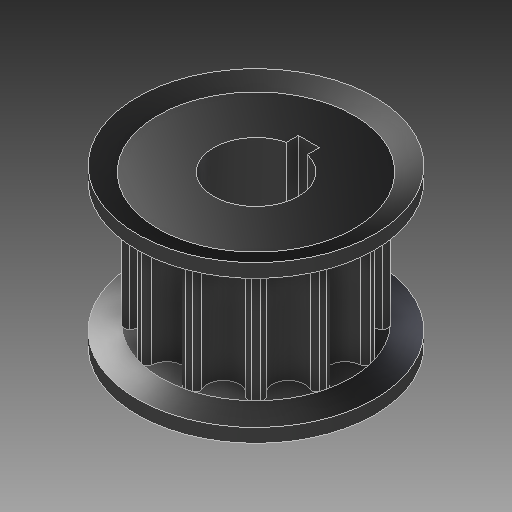
# Autodesk Inventor part: Timing Pulleys
Saved by Autodesk Inventor 2023 (Build 270158000, 158)
## iProperties
Created: 2020-11-14
Material: Nylon 6/6
Document SubType Name: Modeling
Density: 1.13 g/cm^3
Appearance: Glossy - Black
Mass: 24.0165 g
Surface Area: 135.444 cm^2
Volume: 21.2535 cm^3
Revision Number: 0
Autodesk Inventor part; units mm, degrees
ref_plane "YZ Plane" through (0, 0, 0) normal (1, 0, 0) x (0, 1, 0)
ref_plane "XZ Plane" through (0, 0, 0) normal (0, 1, 0) x (-1, 0, 0)
ref_plane "XY Plane" through (0, 0, 0) normal (0, 0, 1) x (1, 0, 0)
sketch "Sketch1" plane through (0, 0, 0) normal (0, 1, 0) x (-1, 0, 0)
  circle A0 centre (0, 0) radius 8.9778
  dimension "d0" = 17.9556
  constraints: 1 centre point, 1 coincident
  measures "d0" diameter of A0
extrude "Extrusion1" add sketch "Sketch1" along normal mid plane 11
sketch "Sketch10" plane through (0, -5.5, 0) normal (0, -1, 0) x (1, 0, 0)
  circle A0 centre (0, 0) radius 8.9778 projected
  circle A1 centre (0, 0) radius 6.9178 construction
  arc A2 (1.5221, -8.3486) -> (-1.5221, -8.3486) centre (0, -8.4428) ccw
  arc A3 (-2.0494, -8.7407) -> (-1.5221, -8.3486) centre (-1.9513, -8.3221) ccw
  line L0 (0, 0) -> (0, -17.4745) construction
  line L1 (0, 0) -> (-8.9342, -15.4745) construction
  circle A4 centre (0, 0) radius 8.9778 projected
  arc A5 (1.5221, -8.3486) -> (2.0494, -8.7407) centre (1.9513, -8.3221) ccw
  point P0 (-2.0494, -8.7407)
  dimension "d62" = 2.06
  dimension "d63" = 3.05
  dimension "d64" = 0.86
  dimension "d65" = 30
  constraints: 8 point on circle, 4 centre point, 4 end point, 3 tangent, 1 symmetric about line, 1 vertical, 1 vertical alignment, 1 other
  measures "d62" radial gap between concentric circles of A0 A1
  measures "d63" diameter of A2
  measures "d64" diameter of A3
  measures "d65" angle of L0 L1
extrude "HTD 5mm Profile" cut sketch "Sketch10" against normal blind 25.4 contours A3 A2 A5 A0 picked at (0.0589, -8.2769)
sketch "Sketch2" plane through (0, 5.5, 0) normal (0, 1, 0) x (1, 0, 0)
  arc A0 (-2.0494, 8.7407) -> (2.0494, 8.7407) centre (0, 0) ccw projected
  arc A1 (-8.8102, -1.0082) -> (-8.9151, -1.0594) centre (-8.7336, -1.298) ccw
  arc A2 (-8.5536, -0.9436) -> (-8.5536, 0.9436) centre (-8.7797, 0) ccw
  arc A3 (-8.9151, 1.0594) -> (-8.8102, 1.0082) centre (-8.7336, 1.298) ccw
  line L0 (0, 0) -> (-21.2101, 0) construction
  arc A4 (-8.5536, -0.9436) -> (-8.8102, -1.0082) centre (-5.8906, -12.059) ccw
  arc A5 (-8.8102, 1.0082) -> (-8.5536, 0.9436) centre (-5.8906, 12.059) ccw
  line L1 (0, 0) -> (0, 6.3397) construction
  line L2 (-8.9778, 0) -> (-8.9778, -190.5824) construction
  arc A6 (-8.9151, 1.0594) -> (-8.9151, -1.0594) centre (0, 0) ccw
  dimension "d3" = 0.9703
  dimension "d5" = 0.2997
  dimension "d7" = 11.43
  dimension "d9" = 7.8094
  dimension "d10" = 8.8102
  dimension "d11" = 8.5536
  dimension "d29" = 0.1676
  dimension "d30" = 0.4242
  dimension "d31" = 1.1684
  constraints: 16 point on circle, 6 centre point, 6 end point, 3 tangent, 2 symmetric about line, 1 horizontal, 1 perpendicular, 1 point on line, 1 vertical, 2 other
  measures "d3" radius of A2
  measures "d5" radius of A3
  measures "d7" radius of A4
  measures "d9" distance edge to line of A2 L1
  measures "d10" distance from line of L1 A3.end
  measures "d11" distance from line of L1 A2.end
  measures "d29" distance from line of A3.end L2
  measures "d30" distance from line of A2.end L2
extrude "GT2 3mm Profile" [suppressed]
pattern_circular "Circular Pattern1" count 12 over 360 about axis through (0, 0, 0) along (0, 1, 0) of "HTD 5mm Profile"
sketch "Sketch7" plane through (0, 0, 0) normal (0, 0, 1) x (1, 0, 0)
  line L0 (8.9778, 5.5) -> (11.2253, 6.1022)
  line L1 (11.2253, 6.1022) -> (11.2253, 7.3976)
  line L2 (11.2253, 7.3976) -> (9.2749, 6.875)
  line L3 (9.2749, 6.875) -> (1.905, 6.875)
  line L4 (1.905, 6.875) -> (1.905, 7.25)
  line L5 (1.905, 7.25) -> (1.5875, 7.25)
  line L6 (1.5875, 7.25) -> (1.5875, 5.5)
  line L7 (0, 5.5) -> (0, 8.7778)
  line L8 (8.9778, 5.5) -> (0, 5.5)
  line L9 (8.9778, 0) -> (-8.9778, 0) projected
  line L10 (1.905, 7.25) -> (11.2253, 7.25)
  line L11 (11.2253, 7.25) -> (11.2253, 7.3976)
  line L12 (0, -1.7556) -> (0, 10.5334) projected
  line L13 (-39.2049, 0) -> (39.2049, 0) projected
  line L14 (-2.0494, 5.5) -> (-2.5955, 5.5) projected
  line L15 (-8.7407, 5.5) -> (-8.5944, 5.5) projected
  line L16 (-6.545, 5.5) -> (-6.1452, 5.5) projected
  line L17 (-2.5955, 5.5) -> (-2.0494, 5.5) projected
  line L18 (2.0494, 5.5) -> (2.5955, 5.5) projected
  line L19 (-6.1452, 5.5) -> (-6.545, 5.5) projected
  line L20 (-8.5944, 5.5) -> (-8.7407, 5.5) projected
  line L21 (6.1452, 5.5) -> (6.545, 5.5) projected
  line L22 (8.5944, 5.5) -> (8.7407, 5.5) projected
  line L23 (8.7407, 5.5) -> (8.5944, 5.5) projected
  line L24 (2.0494, 5.5) -> (1.5221, 5.5) projected
  line L25 (1.5221, 5.5) -> (-1.5221, 5.5) projected
  line L26 (-1.5221, 5.5) -> (-2.0494, 5.5) projected
  line L27 (-2.5955, 5.5) -> (-2.8562, 5.5) projected
  line L28 (-2.8562, 5.5) -> (-5.4925, 5.5) projected
  line L29 (-5.4925, 5.5) -> (-6.1452, 5.5) projected
  line L30 (-6.545, 5.5) -> (-6.4691, 5.5) projected
  line L31 (-6.4691, 5.5) -> (-7.9912, 5.5) projected
  line L32 (-7.9912, 5.5) -> (-8.5944, 5.5) projected
  line L33 (-8.7407, 5.5) -> (-8.3486, 5.5) projected
  line L34 (-8.3486, 5.5) -> (-8.3486, 5.5) projected
  line L35 (-8.3486, 5.5) -> (-8.7407, 5.5) projected
  line L36 (-8.5944, 5.5) -> (-7.9912, 5.5) projected
  line L37 (-7.9912, 5.5) -> (-6.4691, 5.5) projected
  line L38 (-6.4691, 5.5) -> (-6.545, 5.5) projected
  line L39 (-6.1452, 5.5) -> (-5.4925, 5.5) projected
  line L40 (-5.4925, 5.5) -> (-2.8562, 5.5) projected
  line L41 (-2.8562, 5.5) -> (-2.5955, 5.5) projected
  line L42 (-2.0494, 5.5) -> (-1.5221, 5.5) projected
  line L43 (-1.5221, 5.5) -> (1.5221, 5.5) projected
  line L44 (1.5221, 5.5) -> (2.0494, 5.5) projected
  line L45 (2.5955, 5.5) -> (2.8562, 5.5) projected
  line L46 (2.8562, 5.5) -> (5.4925, 5.5) projected
  line L47 (5.4925, 5.5) -> (6.1452, 5.5) projected
  line L48 (6.545, 5.5) -> (6.4691, 5.5) projected
  line L49 (6.4691, 5.5) -> (7.9912, 5.5) projected
  line L50 (7.9912, 5.5) -> (8.5944, 5.5) projected
  line L51 (8.7407, 5.5) -> (8.3486, 5.5) projected
  line L52 (8.3486, 5.5) -> (8.3486, 5.5) projected
  line L53 (8.3486, 5.5) -> (8.7407, 5.5) projected
  line L54 (2.5955, 5.5) -> (2.0494, 5.5) projected
  line L55 (8.5944, 5.5) -> (7.9912, 5.5) projected
  line L56 (7.9912, 5.5) -> (6.4691, 5.5) projected
  line L57 (6.4691, 5.5) -> (6.545, 5.5) projected
  line L58 (6.545, 5.5) -> (6.1452, 5.5) projected
  line L59 (6.1452, 5.5) -> (5.4925, 5.5) projected
  line L60 (5.4925, 5.5) -> (2.8562, 5.5) projected
  line L61 (2.8562, 5.5) -> (2.5955, 5.5) projected
  point P0 (0, 0)
  point P1 (28.0035, 5.334)
  point P2 (-28.0035, 5.334)
  point P3 (0, 5.334)
  point P4 (16.8021, 5.5)
  point P5 (-16.8021, 5.5)
  point P6 (10.6744, 7.25)
  dimension "HexSize" = 3.175
  dimension "BossOD" = 3.81
  dimension "FlangeEdgeThickness" = 1.2954
  dimension "FlangeBaseThickness" = 1.375
  dimension "d41" = 165
  dimension "FlangeStickout" = 2.2475
  dimension "d47" = 17.9556
  dimension "d59" = 5.5
  dimension "HexThickness" = 14.5
  constraints: 22 end point, 4 vertical, 2 horizontal, 2 perpendicular, 1 collinear, 1 parallel, 1 point on line
  measures "HexSize" diameter of L6 L7
  measures "BossOD" diameter of L4 L7
  measures "FlangeEdgeThickness" distance of L0.end L1.end
  measures "FlangeBaseThickness" distance between parallel lines of L8 L3
  measures "d41" angle of L8 L0
  measures "FlangeStickout" horizontal distance of L0.end L0.start
  measures "d47" diameter of L0.start L7
  measures "d59" distance from line of L7.start L13
  measures "HexThickness" diameter of L5 L13
revolve "Revolution1" add sketch "Sketch7" angle 360 about axis through (0, 5.5, 0) along (0, 1, 0) contours L8 L6 L5 L4 L3 L2 L10 L1 L0 | L10 L2 L1
sketch "Sketch9" plane through (0, 6.875, 0) normal (0, 1, 0) x (1, 0, 0)
  circle A0 centre (0, 0) radius 16.89
  circle A1 centre (0, 0) radius 19.5
  circle A2 centre (0, 0) radius 1.905 projected
  dimension "PocketOD" = 39
  dimension "d57" = 2.61
  constraints: 2 centre point, 1 coincident
  measures "PocketOD" diameter of A1
  measures "d57" radial gap between concentric circles of A1 A0
extrude "Extrusion7" [suppressed]
extrude "Extrusion8" [suppressed]
revolve "3D Printed Revolve" [suppressed]
sketch "Sketch16" plane through (0, 0, 0) normal (1, 0, 0) x (0, 1, 0)
  line L0 (6.875, 9.2749) -> (6.875, -9.2749) projected
  line L1 (7.25, 1.5875) -> (7.25, -1.5875) projected
  line L2 (6.875, 1.5875) -> (7.6116, 1.5875)
  line L3 (6.875, -1.5875) -> (7.6116, -1.5875)
  line L4 (6.875, 1.5875) -> (6.875, 6.3881)
  line L5 (6.875, 6.3881) -> (7.6116, 6.3881)
  line L6 (7.6116, 6.3881) -> (7.6116, 1.5875)
  line L7 (6.875, -1.5875) -> (6.875, -6.3881)
  line L8 (6.875, -6.3881) -> (7.6116, -6.3881)
  line L9 (7.6116, -6.3881) -> (7.6116, -1.5875)
  line L10 (-1.5223, 0) -> (9.1339, 0) projected
  point P0 (0, 0)
  point P1 (6.5, 8.89)
  point P2 (6.5, -8.89)
  point P3 (6.5, 7.3131)
  point P4 (6.875, 6.3881)
  point P5 (6.875, 6.35)
  dimension "RaiseHt" = 0.7366
  dimension "RaiseOd" = 12.7762
  constraints: 16 end point, 6 point on line, 3 horizontal, 3 perpendicular, 1 collinear, 1 vertical alignment
  measures "RaiseHt" distance of L4.end L5.end
  measures "RaiseOd" distance between parallel lines of L5 L8
revolve "EndRaise" [suppressed]
mirror "Mirror2" about plane through (0, 0, 0) normal (0, 1, 0) of "Revolution1"
fillet "Fillet1" [suppressed]
sketch "Sketch8" plane through (0, 7.25, 0) normal (0, 1, 0) x (1, 0, 0)
  circle A0 centre (0, 0) radius 1.5875 projected
  line L0 (-1.8331, 0) -> (-0.9165, 1.5875)
  line L1 (-0.9165, 1.5875) -> (0.9165, 1.5875)
  line L2 (0.9165, 1.5875) -> (1.8331, 0)
  line L3 (1.8331, 0) -> (0.9165, -1.5875)
  line L4 (0.9165, -1.5875) -> (-0.9165, -1.5875)
  line L5 (-0.9165, -1.5875) -> (-1.8331, 0)
  constraints: 12 end point, 1 coincident, 1 horizontal, 1 tangent, 13 other
extrude "Hex Bore" [suppressed]
sketch "Sketch12" plane through (0, 0, 0) normal (1, 0, 0) x (0, 1, 0)
  line L0 (13.7296, 5.5563) -> (6.8716, 5.5563)
  line L1 (6.8716, 5.5563) -> (6.8716, 1.5875)
  line L2 (6.8716, 1.5875) -> (7.3796, 1.5875)
  line L3 (7.3796, 1.5875) -> (7.3796, 4)
  line L4 (7.3796, 4) -> (13.7296, 4)
  line L5 (13.7296, 4) -> (13.7296, 5.5563)
  line L6 (-2.7459, 0) -> (16.4755, 0) projected
  point P0 (0, 0)
  dimension "d103" = 1.5875
  dimension "d104" = 6.8716
  dimension "d105" = 5.5563
  dimension "d106" = 4
  dimension "d107" = 0.508
  dimension "d108" = 6.858
  constraints: 12 end point, 5 perpendicular, 1 horizontal
  measures "d103" distance from line of point (0, 0) L2
  measures "d104" distance from line of point (0, 0) L1
  measures "d105" distance from line of point (0, 0) L0
  measures "d106" distance from line of point (0, 0) L4
  measures "d107" distance between parallel lines of L1 L3
  measures "d108" distance between parallel lines of L1 L5
revolve "SetScrewRevolve" [suppressed]
sketch "Sketch13" plane through (0, 0, 0) normal (1, 0, 0) x (0, 1, 0)
  circle A0 centre (11, 0) radius 2.0828
  line L0 (14.175, -9.6338) -> (14.175, 9.6338)
  point P0 (0, 0)
  dimension "d76" = 4.1656
  dimension "d92" = 3.175
  dimension "d100" = 11
  constraints: 2 end point, 1 centre point, 1 horizontal alignment
  measures "d76" diameter of A0
  measures "d92" distance from line of L0 A0.centre
  measures "d100" distance of point (0, 0) A0.centre
extrude "SetScrewHole" [suppressed]
sketch "Sketch14" plane through (0, 0, 0) normal (0, 1, 0) x (-1, 0, 0)
  circle A0 centre (0, 0) radius 3
  line L0 (-1.6583, -2.5) -> (1.6583, -2.5)
  dimension "d83" = 6
  dimension "d84" = 2.5
  constraints: 2 end point, 2 point on circle, 1 centre point, 1 coincident, 1 horizontal
  measures "d83" diameter of A0
  measures "d84" distance from line of L0 point (0, 0)
extrude "D-Shaft" [suppressed]
sketch "Sketch15" plane through (0, 0, 0) normal (0, 1, 0) x (-1, 0, 0)
  circle A0 centre (0, 0) radius 4
  line L0 (1, 5) -> (-1, 5)
  line L1 (-1, 5) -> (-1, -5)
  line L2 (-1, -5) -> (1, -5)
  line L3 (1, -5) -> (1, 5)
  line L4 (1, 5) -> (-1, -5) construction
  line L5 (-1, 5) -> (1, -5) construction
  point P0 (-1, -3.873)
  point P1 (1, -3.873)
  dimension "d87" = 8
  dimension "d88" = 2
  dimension "d89" = 10
  constraints: 12 end point, 2 midpoint, 2 parallel, 1 centre point, 1 coincident, 1 horizontal, 1 perpendicular
  measures "d87" diameter of A0
  measures "d88" distance of L2.end L1.end
  measures "d89" distance of L1.end L0.end
extrude "Cim Shaft" cut sketch "Sketch15" against normal through all both and the other way through all contours A0 L3 | L3 A0 L1 | L3 L2 L1 A0 | L1 A0
sketch "Sketch17" plane through (0, 0, 0) normal (0, 1, 0) x (-1, 0, 0)
  circle A0 centre (0, 0) radius 1.5875
  dimension "MotorHoleOD" = 3.175
  constraints: 1 centre point, 1 coincident
  measures "MotorHoleOD" diameter of A0
extrude "MotorHole" [suppressed]
equation "\"Teeth\" = 12"
equation "\"d47\" = d0"
body "Solid1"
